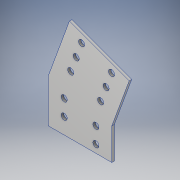
# Autodesk Inventor part: ARM_071_TwoPieceIntakeGusset
Saved by Autodesk Inventor 2018.3 (Build 223284000, 284)
## iProperties
Created: 2020-02-12
Part Number: ARM_071_TwoPieceIntakeGusset
Material: Aluminum 6061
Document SubType Name: Modeling
Designer: 22barlalex
Density: 2.7 g/cm^3
Appearance: Aluminum - Flat
Author: 22barlalex
Autodesk Inventor part; units mm, degrees
ref_plane "YZ Plane" through (0, 0, 0) normal (1, 0, 0) x (0, 1, 0)
ref_plane "XZ Plane" through (0, 0, 0) normal (0, 1, 0) x (-1, 0, 0)
ref_plane "XY Plane" through (0, 0, 0) normal (0, 0, 1) x (1, 0, 0)
sketch "Sketch1" plane through (0, 0, 0) normal (0, 0, 1) x (1, 0, 0)
  line L0 (0, 0) -> (50.8, 0)
  line L1 (50.8, 0) -> (50.8, 25.4)
  line L2 (50.8, 25.4) -> (64.6673, 63.5)
  line L3 (64.6673, 63.5) -> (16.8775, 80.8941)
  line L4 (16.8775, 80.8941) -> (0, 34.5237)
  line L5 (0, 34.5237) -> (0, 0)
  line L6 (0, 34.5237) -> (50.8, 25.4) construction
  dimension "d0" = 50.8
  dimension "d1" = 160
  dimension "d2" = 25.4
  dimension "d3" = 51.6128
  dimension "d4" = 38.1
  constraints: 14 end point, 2 parallel, 2 perpendicular, 1 horizontal
  measures "d0" distance of L0.start L0.end
  measures "d1" angle of L1 L2
  measures "d2" distance of L0.end L1.end
  measures "d3" distance of L4.end L1.end
  measures "d4" vertical distance of L2.end L1.end
extrude "Extrusion1" add sketch "Sketch1" along normal blind 2.032
sketch "Sketch2" plane through (0, 0, 2.032) normal (0, 0, 1) x (1, 0, 0)
  line L0 (0, 0) -> (50.8, 0) projected
  line L1 (50.8, 0) -> (50.8, 25.4) projected
  line L2 (50.8, 25.4) -> (64.6673, 63.5) projected
  line L3 (64.6673, 63.5) -> (16.8775, 80.8941) projected
  line L4 (16.8775, 80.8941) -> (0, 34.5237) projected
  line L5 (0, 34.5237) -> (0, 0) projected
  point P0 (41.874, 38.0084)
  point P1 (46.2177, 49.9425)
  point P2 (50.5613, 61.8766)
  point P3 (17.9524, 46.7152)
  point P4 (22.2961, 58.6493)
  point P5 (26.6397, 70.5834)
  point P6 (38.1, 6.35)
  point P7 (38.1, 19.05)
  point P8 (12.7, 25.4)
  point P9 (12.7, 12.7)
  dimension "d14" = 12.7
  dimension "d15" = 12.7
  dimension "d16" = 12.7
  dimension "d17" = 6.35
  dimension "d18" = 12.7
  dimension "d19" = 12.7
  dimension "d20" = 12.7
  dimension "d21" = 12.7
  dimension "d22" = 12.7
  dimension "d23" = 6.35
  dimension "d24" = 12.7
  dimension "d25" = 12.7
  dimension "d33" = 12.7
  dimension "d34" = 12.7
  dimension "d35" = 6.35
  dimension "d36" = 12.7
  dimension "d37" = 12.7
  dimension "d38" = 12.7
  constraints: 2 vertical alignment
  measures "d14" distance from line of L2 point (50.561, 61.877)
  measures "d15" distance from line of L2 point (46.218, 49.943)
  measures "d16" distance from line of L2 point (41.874, 38.008)
  measures "d17" distance from line of L3 point (50.561, 61.877)
  measures "d18" distance of point (50.561, 61.877) point (46.218, 49.943)
  measures "d19" distance of point (46.218, 49.943) point (41.874, 38.008)
  measures "d20" distance from line of L4 point (26.64, 70.583)
  measures "d21" distance from line of L4 point (22.296, 58.649)
  measures "d22" distance from line of L4 point (17.952, 46.715)
  measures "d23" distance from line of L3 point (26.64, 70.583)
  measures "d24" distance of point (26.64, 70.583) point (22.296, 58.649)
  measures "d25" distance of point (22.296, 58.649) point (17.952, 46.715)
  measures "d33" distance from line of L5 point (12.7, 25.4)
  measures "d34" distance from line of L1 point (38.1, 19.05)
  measures "d35" distance from line of L0 point (38.1, 6.35)
  measures "d36" distance of point (38.1, 19.05) point (38.1, 6.35)
  measures "d37" distance from line of L0 point (12.7, 12.7)
  measures "d38" distance of point (12.7, 25.4) point (12.7, 12.7)
hole "Hole2" at (41.874, 38.0084, 2.032) at (46.2177, 49.9425, 2.032) at (50.5613, 61.8766, 2.032) at (17.9524, 46.7152, 2.032) at (22.2961, 58.6493, 2.032) at (26.6397, 70.5834, 2.032) at (38.1, 6.35, 2.032) at (38.1, 19.05, 2.032) at (12.7, 25.4, 2.032) at (12.7, 12.7, 2.032) direction (0, 0, -1) diameter 4.8514 end through all
body "Solid1"
